Autodesk Inventor part; units mm, degrees
(part 3 of 3)
sketch "Sketch5" plane through (203.2, 0, 0) normal (0, 0, -1) x (-1, 0, 0)
  line L0 (0, 0) -> (203.2, 0) projected
  line L1 (0, 0) -> (0, -25.4) projected
  line L2 (203.2, -25.4) -> (0, -25.4) projected
  line L3 (203.2, 0) -> (203.2, -25.4) projected
  line L4 (18.6693, -4.254) -> (184.5307, -4.254) construction
  line L5 (184.5307, -4.254) -> (184.5307, -21.146) construction
  line L6 (184.5307, -21.146) -> (18.6693, -21.146) construction
  line L7 (18.6693, -21.146) -> (18.6693, -4.254) construction
  spline S0 degree 2 poles (29.2483, -14.4636) (29.2483, -15.1453) (28.7296, -16.1901) (28.2998, -16.531) knots 0 0 0 1 2 2 2
  spline S1 degree 2 poles (28.2998, -16.531) (27.7811, -16.9311) (26.6029, -17.272) (25.6692, -17.272) knots 0 0 0 1 2 2 2
  line L8 (25.6692, -17.272) -> (23.0461, -17.272)
  line L9 (23.0461, -17.272) -> (23.0461, -8.128)
  line L10 (23.0461, -8.128) -> (25.4692, -8.128)
  spline S2 degree 2 poles (25.4692, -8.128) (26.4473, -8.128) (27.4254, -8.254) (27.87, -8.4985) knots 0 0 0 1 2 2 2
  spline S3 degree 2 poles (27.87, -8.4985) (28.3665, -8.7579) (28.8185, -9.61) (28.8185, -10.188) knots 0 0 0 1 2 2 2
  spline S4 degree 2 poles (28.8185, -10.188) (28.8185, -10.8327) (28.1368, -11.8553) (27.5366, -12.1442) knots 0 0 0 1 2 2 2
  line L11 (27.5366, -12.1442) -> (27.5366, -12.1887)
  spline S5 degree 2 poles (27.5366, -12.1887) (28.3517, -12.411) (29.2483, -13.5892) (29.2483, -14.4636) knots 0 0 0 1 2 2 2
  spline S6 degree 2 poles (27.9812, -14.5155) (27.9812, -13.9968) (27.6848, -13.3299) (27.2402, -13.0927) knots 0 0 0 1 2 2 2
  spline S7 degree 2 poles (27.2402, -13.0927) (26.9512, -12.9445) (26.2694, -12.8556) (25.6396, -12.8556) knots 0 0 0 1 2 2 2
  line L12 (25.6396, -12.8556) -> (24.2613, -12.8556)
  line L13 (24.2613, -12.8556) -> (24.2613, -16.2346)
  line L14 (24.2613, -16.2346) -> (25.2469, -16.2346)
  spline S8 degree 2 poles (25.2469, -16.2346) (26.0471, -16.2346) (26.966, -16.0864) (27.3217, -15.8493) knots 0 0 0 1 2 2 2
  spline S9 degree 2 poles (27.3217, -15.8493) (27.6625, -15.6047) (27.9812, -14.9971) (27.9812, -14.5155) knots 0 0 0 1 2 2 2
  spline S10 degree 2 poles (27.5514, -10.3584) (27.5514, -10.0324) (27.3291, -9.5433) (27.0846, -9.4025) knots 0 0 0 1 2 2 2
  spline S11 degree 2 poles (27.0846, -9.4025) (26.7882, -9.2395) (26.0694, -9.1654) (25.4247, -9.1654) knots 0 0 0 1 2 2 2
  line L15 (25.4247, -9.1654) -> (24.2613, -9.1654)
  line L16 (24.2613, -9.1654) -> (24.2613, -11.8404)
  line L17 (24.2613, -11.8404) -> (25.6396, -11.8404)
  spline S12 degree 2 poles (25.6396, -11.8404) (26.2102, -11.8404) (26.7511, -11.7219) (27.0401, -11.5366) knots 0 0 0 1 2 2 2
  spline S13 degree 2 poles (27.0401, -11.5366) (27.3217, -11.3588) (27.5514, -10.7882) (27.5514, -10.3584) knots 0 0 0 1 2 2 2
  line L18 (29.4706, -17.272) -> (32.5532, -8.128)
  line L19 (32.5532, -8.128) -> (34.05, -8.128)
  line L20 (34.05, -8.128) -> (37.1326, -17.272)
  line L21 (37.1326, -17.272) -> (35.8506, -17.272)
  line L22 (35.8506, -17.272) -> (35.0207, -14.7155)
  line L23 (35.0207, -14.7155) -> (31.5306, -14.7155)
  line L24 (31.5306, -14.7155) -> (30.7007, -17.272)
  line L25 (30.7007, -17.272) -> (29.4706, -17.272)
  line L26 (34.6873, -13.6781) -> (33.2719, -9.3729)
  line L27 (33.2719, -9.3729) -> (31.864, -13.6781)
  line L28 (31.864, -13.6781) -> (34.6873, -13.6781)
  spline S14 degree 2 poles (40.5486, -17.435) (39.5557, -17.435) (38.1626, -17.0201) (37.5475, -16.7237) knots 0 0 0 1 2 2 2
  line L29 (37.5475, -16.7237) -> (37.5475, -15.1972)
  line L30 (37.5475, -15.1972) -> (37.6365, -15.1972)
  spline S15 degree 2 poles (37.6365, -15.1972) (38.2367, -15.7604) (39.7557, -16.3828) (40.4597, -16.3828) knots 0 0 0 1 2 2 2
  spline S16 degree 2 poles (40.4597, -16.3828) (41.4675, -16.3828) (42.4975, -15.5455) (42.4975, -14.8563) knots 0 0 0 1 2 2 2
  spline S17 degree 2 poles (42.4975, -14.8563) (42.4975, -14.308) (41.9565, -13.6263) (41.3711, -13.4558) knots 0 0 0 1 2 2 2
  spline S18 degree 2 poles (41.3711, -13.4558) (40.9488, -13.3373) (40.2448, -13.1742) (39.7187, -13.0409) knots 0 0 0 1 2 2 2
  spline S19 degree 2 poles (39.7187, -13.0409) (39.2444, -12.9149) (38.496, -12.537) (38.207, -12.2332) knots 0 0 0 1 2 2 2
  spline S20 degree 2 poles (38.207, -12.2332) (37.9255, -11.9294) (37.6142, -11.1142) (37.6142, -10.5807) knots 0 0 0 1 2 2 2
  spline S21 degree 2 poles (37.6142, -10.5807) (37.6142, -9.4692) (39.3482, -7.965) (40.6894, -7.965) knots 0 0 0 1 2 2 2
  spline S22 degree 2 poles (40.6894, -7.965) (41.46, -7.965) (42.8235, -8.2688) (43.4089, -8.5578) knots 0 0 0 1 2 2 2
  line L31 (43.4089, -8.5578) -> (43.4089, -10.0102)
  line L32 (43.4089, -10.0102) -> (43.32, -10.0102)
  spline S23 degree 2 poles (43.32, -10.0102) (42.8828, -9.61) (41.5193, -9.0172) (40.7709, -9.0172) knots 0 0 0 1 2 2 2
  spline S24 degree 2 poles (40.7709, -9.0172) (39.9262, -9.0172) (38.8814, -9.8101) (38.8814, -10.4548) knots 0 0 0 1 2 2 2
  spline S25 degree 2 poles (38.8814, -10.4548) (38.8814, -11.0327) (39.4964, -11.7219) (40.0744, -11.8775) knots 0 0 0 1 2 2 2
  spline S26 degree 2 poles (40.0744, -11.8775) (40.4597, -11.9812) (41.5786, -12.248) (41.9491, -12.3591) knots 0 0 0 1 2 2 2
  spline S27 degree 2 poles (41.9491, -12.3591) (42.8902, -12.6481) (43.7646, -13.8115) (43.7646, -14.6637) knots 0 0 0 1 2 2 2
  spline S28 degree 2 poles (43.7646, -14.6637) (43.7646, -15.2046) (43.3274, -16.242) (42.9346, -16.6051) knots 0 0 0 1 2 2 2
  spline S29 degree 2 poles (42.9346, -16.6051) (42.4975, -17.0052) (41.3859, -17.435) (40.5486, -17.435) knots 0 0 0 1 2 2 2
  line L33 (45.0021, -17.272) -> (45.0021, -8.128)
  line L34 (45.0021, -8.128) -> (50.7226, -8.128)
  line L35 (50.7226, -8.128) -> (50.7226, -9.2099)
  line L36 (50.7226, -9.2099) -> (46.2173, -9.2099)
  line L37 (46.2173, -9.2099) -> (46.2173, -11.7145)
  line L38 (46.2173, -11.7145) -> (50.4188, -11.7145)
  line L39 (50.4188, -11.7145) -> (50.4188, -12.7963)
  line L40 (50.4188, -12.7963) -> (46.2173, -12.7963)
  line L41 (46.2173, -12.7963) -> (46.2173, -16.1901)
  line L42 (46.2173, -16.1901) -> (50.7226, -16.1901)
  line L43 (50.7226, -16.1901) -> (50.7226, -17.272)
  line L44 (50.7226, -17.272) -> (45.0021, -17.272)
  line L45 (61.4524, -9.2099) -> (57.199, -9.2099)
  line L46 (57.199, -9.2099) -> (57.199, -11.7886)
  line L47 (57.199, -11.7886) -> (61.2745, -11.7886)
  line L48 (61.2745, -11.7886) -> (61.2745, -12.8704)
  line L49 (61.2745, -12.8704) -> (57.199, -12.8704)
  line L50 (57.199, -12.8704) -> (57.199, -17.272)
  line L51 (57.199, -17.272) -> (55.9837, -17.272)
  line L52 (55.9837, -17.272) -> (55.9837, -8.128)
  line L53 (55.9837, -8.128) -> (61.4524, -8.128)
  line L54 (61.4524, -8.128) -> (61.4524, -9.2099)
  spline S30 degree 2 poles (69.0106, -9.1728) (69.5293, -9.7804) (70.1073, -11.5589) (70.1073, -12.7) knots 0 0 0 1 2 2 2
  spline S31 degree 2 poles (70.1073, -12.7) (70.1073, -13.8115) (69.5441, -15.6121) (69.0106, -16.2198) knots 0 0 0 1 2 2 2
  spline S32 degree 2 poles (69.0106, -16.2198) (68.4474, -16.857) (66.958, -17.4647) (66.0614, -17.4647) knots 0 0 0 1 2 2 2
  spline S33 degree 2 poles (66.0614, -17.4647) (65.1352, -17.4647) (63.6531, -16.8348) (63.1122, -16.2198) knots 0 0 0 1 2 2 2
  spline S34 degree 2 poles (63.1122, -16.2198) (62.5861, -15.6121) (62.0229, -13.8263) (62.0229, -12.7) knots 0 0 0 1 2 2 2
  spline S35 degree 2 poles (62.0229, -12.7) (62.0229, -11.5514) (62.5935, -9.8027) (63.1196, -9.1728) knots 0 0 0 1 2 2 2
  spline S36 degree 2 poles (63.1196, -9.1728) (63.6531, -8.5652) (65.1426, -7.9353) (66.0614, -7.9353) knots 0 0 0 1 2 2 2
  spline S37 degree 2 poles (66.0614, -7.9353) (66.9951, -7.9353) (68.4919, -8.5874) (69.0106, -9.1728) knots 0 0 0 1 2 2 2
  spline S38 degree 2 poles (68.8402, -12.7) (68.8402, -11.796) (68.4474, -10.3955) (68.0918, -9.9361) knots 0 0 0 1 2 2 2
  spline S39 degree 2 poles (68.0918, -9.9361) (67.7287, -9.4618) (66.7061, -8.9876) (66.0688, -8.9876) knots 0 0 0 1 2 2 2
  spline S40 degree 2 poles (66.0688, -8.9876) (65.4093, -8.9876) (64.4164, -9.447) (64.0385, -9.9361) knots 0 0 0 1 2 2 2
  spline S41 degree 2 poles (64.0385, -9.9361) (63.6754, -10.4029) (63.2901, -11.8108) (63.2901, -12.7) knots 0 0 0 1 2 2 2
  spline S42 degree 2 poles (63.2901, -12.7) (63.2901, -14.5006) (64.8017, -16.4124) (66.0688, -16.4124) knots 0 0 0 1 2 2 2
  spline S43 degree 2 poles (66.0688, -16.4124) (67.3359, -16.4124) (68.8402, -14.5006) (68.8402, -12.7) knots 0 0 0 1 2 2 2
  spline S44 degree 2 poles (74.6348, -17.4647) (73.8271, -17.4647) (72.6267, -17.0423) (72.2043, -16.6199) knots 0 0 0 1 2 2 2
  spline S45 degree 2 poles (72.2043, -16.6199) (71.7227, -16.1457) (71.33, -14.8119) (71.33, -13.8337) knots 0 0 0 1 2 2 2
  line L55 (71.33, -13.8337) -> (71.33, -8.128)
  line L56 (71.33, -8.128) -> (72.5452, -8.128)
  line L57 (72.5452, -8.128) -> (72.5452, -13.8337)
  spline S46 degree 2 poles (72.5452, -13.8337) (72.5452, -14.471) (72.7082, -15.3306) (72.9379, -15.6788) knots 0 0 0 1 2 2 2
  spline S47 degree 2 poles (72.9379, -15.6788) (73.1825, -16.0493) (74.0272, -16.4273) (74.6348, -16.4273) knots 0 0 0 1 2 2 2
  spline S48 degree 2 poles (74.6348, -16.4273) (75.2054, -16.4273) (76.0946, -16.0493) (76.3391, -15.6788) knots 0 0 0 1 2 2 2
  spline S49 degree 2 poles (76.3391, -15.6788) (76.5689, -15.3306) (76.7319, -14.4784) (76.7319, -13.8634) knots 0 0 0 1 2 2 2
  line L58 (76.7319, -13.8634) -> (76.7319, -8.128)
  line L59 (76.7319, -8.128) -> (77.9471, -8.128)
  line L60 (77.9471, -8.128) -> (77.9471, -13.8337)
  spline S50 degree 2 poles (77.9471, -13.8337) (77.9471, -14.7896) (77.5618, -16.1531) (77.0727, -16.6199) knots 0 0 0 1 2 2 2
  spline S51 degree 2 poles (77.0727, -16.6199) (76.6355, -17.0497) (75.4796, -17.4647) (74.6348, -17.4647) knots 0 0 0 1 2 2 2
  line L61 (86.7651, -17.272) -> (85.1867, -17.272)
  line L62 (85.1867, -17.272) -> (82.2968, -13.6337)
  line L63 (82.2968, -13.6337) -> (80.9037, -13.6337)
  line L64 (80.9037, -13.6337) -> (80.9037, -17.272)
  line L65 (80.9037, -17.272) -> (79.6885, -17.272)
  line L66 (79.6885, -17.272) -> (79.6885, -8.128)
  line L67 (79.6885, -8.128) -> (82.0449, -8.128)
  spline S52 degree 2 poles (82.0449, -8.128) (82.8303, -8.128) (83.89, -8.2984) (84.3716, -8.6097) knots 0 0 0 1 2 2 2
  spline S53 degree 2 poles (84.3716, -8.6097) (84.8533, -8.9209) (85.409, -9.8916) (85.409, -10.6104) knots 0 0 0 1 2 2 2
  spline S54 degree 2 poles (85.409, -10.6104) (85.409, -11.6107) (84.3865, -12.9668) (83.5121, -13.2928) knots 0 0 0 1 2 2 2
  line L68 (83.5121, -13.2928) -> (86.7651, -17.272)
  spline S55 degree 2 poles (84.1419, -10.7067) (84.1419, -10.3066) (83.8603, -9.6915) (83.5639, -9.4914) knots 0 0 0 1 2 2 2
  spline S56 degree 2 poles (83.5639, -9.4914) (83.3046, -9.321) (82.6155, -9.1802) (82.1116, -9.1802) knots 0 0 0 1 2 2 2
  line L69 (82.1116, -9.1802) -> (80.9037, -9.1802)
  line L70 (80.9037, -9.1802) -> (80.9037, -12.6185)
  line L71 (80.9037, -12.6185) -> (81.9708, -12.6185)
  spline S57 degree 2 poles (81.9708, -12.6185) (82.4969, -12.6185) (83.3342, -12.4332) (83.6232, -12.1442) knots 0 0 0 1 2 2 2
  spline S58 degree 2 poles (83.6232, -12.1442) (83.89, -11.8923) (84.1419, -11.1809) (84.1419, -10.7067) knots 0 0 0 1 2 2 2
  line L72 (90.6776, -17.272) -> (87.1356, -17.272)
  line L73 (87.1356, -17.272) -> (87.1356, -16.3383)
  line L74 (87.1356, -16.3383) -> (88.299, -16.3383)
  line L75 (88.299, -16.3383) -> (88.299, -9.0617)
  line L76 (88.299, -9.0617) -> (87.1356, -9.0617)
  line L77 (87.1356, -9.0617) -> (87.1356, -8.128)
  line L78 (87.1356, -8.128) -> (90.6776, -8.128)
  line L79 (90.6776, -8.128) -> (90.6776, -9.0617)
  line L80 (90.6776, -9.0617) -> (89.5142, -9.0617)
  line L81 (89.5142, -9.0617) -> (89.5142, -16.3383)
  line L82 (89.5142, -16.3383) -> (90.6776, -16.3383)
  line L83 (90.6776, -16.3383) -> (90.6776, -17.272)
  line L84 (92.1818, -17.272) -> (92.1818, -8.128)
  line L85 (92.1818, -8.128) -> (97.9024, -8.128)
  line L86 (97.9024, -8.128) -> (97.9024, -9.2099)
  line L87 (97.9024, -9.2099) -> (93.3971, -9.2099)
  line L88 (93.3971, -9.2099) -> (93.3971, -11.7145)
  line L89 (93.3971, -11.7145) -> (97.5986, -11.7145)
  line L90 (97.5986, -11.7145) -> (97.5986, -12.7963)
  line L91 (97.5986, -12.7963) -> (93.3971, -12.7963)
  line L92 (93.3971, -12.7963) -> (93.3971, -16.1901)
  line L93 (93.3971, -16.1901) -> (97.9024, -16.1901)
  line L94 (97.9024, -16.1901) -> (97.9024, -17.272)
  line L95 (97.9024, -17.272) -> (92.1818, -17.272)
  line L96 (106.3128, -17.272) -> (104.7345, -17.272)
  line L97 (104.7345, -17.272) -> (101.8445, -13.6337)
  line L98 (101.8445, -13.6337) -> (100.4514, -13.6337)
  line L99 (100.4514, -13.6337) -> (100.4514, -17.272)
  line L100 (100.4514, -17.272) -> (99.2362, -17.272)
  line L101 (99.2362, -17.272) -> (99.2362, -8.128)
  line L102 (99.2362, -8.128) -> (101.5926, -8.128)
  spline S59 degree 2 poles (101.5926, -8.128) (102.3781, -8.128) (103.4377, -8.2984) (103.9193, -8.6097) knots 0 0 0 1 2 2 2
  spline S60 degree 2 poles (103.9193, -8.6097) (104.401, -8.9209) (104.9568, -9.8916) (104.9568, -10.6104) knots 0 0 0 1 2 2 2
  spline S61 degree 2 poles (104.9568, -10.6104) (104.9568, -11.6107) (103.9342, -12.9668) (103.0598, -13.2928) knots 0 0 0 1 2 2 2
  line L103 (103.0598, -13.2928) -> (106.3128, -17.272)
  spline S62 degree 2 poles (103.6896, -10.7067) (103.6896, -10.3066) (103.4081, -9.6915) (103.1117, -9.4914) knots 0 0 0 1 2 2 2
  spline S63 degree 2 poles (103.1117, -9.4914) (102.8523, -9.321) (102.1632, -9.1802) (101.6593, -9.1802) knots 0 0 0 1 2 2 2
  line L104 (101.6593, -9.1802) -> (100.4514, -9.1802)
  line L105 (100.4514, -9.1802) -> (100.4514, -12.6185)
  line L106 (100.4514, -12.6185) -> (101.5185, -12.6185)
  spline S64 degree 2 poles (101.5185, -12.6185) (102.0446, -12.6185) (102.8819, -12.4332) (103.1709, -12.1442) knots 0 0 0 1 2 2 2
  spline S65 degree 2 poles (103.1709, -12.1442) (103.4377, -11.8923) (103.6896, -11.1809) (103.6896, -10.7067) knots 0 0 0 1 2 2 2
  line L107 (113.1004, -17.272) -> (113.1004, -9.2099)
  line L108 (113.1004, -9.2099) -> (110.0326, -9.2099)
  line L109 (110.0326, -9.2099) -> (110.0326, -8.128)
  line L110 (110.0326, -8.128) -> (117.3834, -8.128)
  line L111 (117.3834, -8.128) -> (117.3834, -9.2099)
  line L112 (117.3834, -9.2099) -> (114.3156, -9.2099)
  line L113 (114.3156, -9.2099) -> (114.3156, -17.272)
  line L114 (114.3156, -17.272) -> (113.1004, -17.272)
  line L115 (125.3863, -17.272) -> (123.8079, -17.272)
  line L116 (123.8079, -17.272) -> (120.918, -13.6337)
  line L117 (120.918, -13.6337) -> (119.5249, -13.6337)
  line L118 (119.5249, -13.6337) -> (119.5249, -17.272)
  line L119 (119.5249, -17.272) -> (118.3097, -17.272)
  line L120 (118.3097, -17.272) -> (118.3097, -8.128)
  line L121 (118.3097, -8.128) -> (120.6661, -8.128)
  spline S66 degree 2 poles (120.6661, -8.128) (121.4515, -8.128) (122.5112, -8.2984) (122.9928, -8.6097) knots 0 0 0 1 2 2 2
  spline S67 degree 2 poles (122.9928, -8.6097) (123.4745, -8.9209) (124.0302, -9.8916) (124.0302, -10.6104) knots 0 0 0 1 2 2 2
  spline S68 degree 2 poles (124.0302, -10.6104) (124.0302, -11.6107) (123.0076, -12.9668) (122.1332, -13.2928) knots 0 0 0 1 2 2 2
  line L122 (122.1332, -13.2928) -> (125.3863, -17.272)
  spline S69 degree 2 poles (122.7631, -10.7067) (122.7631, -10.3066) (122.4815, -9.6915) (122.1851, -9.4914) knots 0 0 0 1 2 2 2
  spline S70 degree 2 poles (122.1851, -9.4914) (121.9258, -9.321) (121.2366, -9.1802) (120.7327, -9.1802) knots 0 0 0 1 2 2 2
  line L123 (120.7327, -9.1802) -> (119.5249, -9.1802)
  line L124 (119.5249, -9.1802) -> (119.5249, -12.6185)
  line L125 (119.5249, -12.6185) -> (120.592, -12.6185)
  spline S71 degree 2 poles (120.592, -12.6185) (121.1181, -12.6185) (121.9554, -12.4332) (122.2444, -12.1442) knots 0 0 0 1 2 2 2
  spline S72 degree 2 poles (122.2444, -12.1442) (122.5112, -11.8923) (122.7631, -11.1809) (122.7631, -10.7067) knots 0 0 0 1 2 2 2
  line L126 (125.1269, -17.272) -> (128.2095, -8.128)
  line L127 (128.2095, -8.128) -> (129.7063, -8.128)
  line L128 (129.7063, -8.128) -> (132.7889, -17.272)
  line L129 (132.7889, -17.272) -> (131.507, -17.272)
  line L130 (131.507, -17.272) -> (130.677, -14.7155)
  line L131 (130.677, -14.7155) -> (127.1869, -14.7155)
  line L132 (127.1869, -14.7155) -> (126.357, -17.272)
  line L133 (126.357, -17.272) -> (125.1269, -17.272)
  line L134 (130.3436, -13.6781) -> (128.9283, -9.3729)
  line L135 (128.9283, -9.3729) -> (127.5204, -13.6781)
  line L136 (127.5204, -13.6781) -> (130.3436, -13.6781)
  line L137 (140.1989, -17.272) -> (138.8355, -17.272)
  line L138 (138.8355, -17.272) -> (134.7896, -9.3877)
  line L139 (134.7896, -9.3877) -> (134.7896, -17.272)
  line L140 (134.7896, -17.272) -> (133.6559, -17.272)
  line L141 (133.6559, -17.272) -> (133.6559, -8.128)
  line L142 (133.6559, -8.128) -> (135.3824, -8.128)
  line L143 (135.3824, -8.128) -> (139.0652, -15.3676)
  line L144 (139.0652, -15.3676) -> (139.0652, -8.128)
  line L145 (139.0652, -8.128) -> (140.1989, -8.128)
  line L146 (140.1989, -8.128) -> (140.1989, -17.272)
  spline S73 degree 2 poles (144.6005, -17.435) (143.6076, -17.435) (142.2145, -17.0201) (141.5994, -16.7237) knots 0 0 0 1 2 2 2
  line L147 (141.5994, -16.7237) -> (141.5994, -15.1972)
  line L148 (141.5994, -15.1972) -> (141.6884, -15.1972)
  spline S74 degree 2 poles (141.6884, -15.1972) (142.2886, -15.7604) (143.8076, -16.3828) (144.5116, -16.3828) knots 0 0 0 1 2 2 2
  spline S75 degree 2 poles (144.5116, -16.3828) (145.5194, -16.3828) (146.5494, -15.5455) (146.5494, -14.8563) knots 0 0 0 1 2 2 2
  spline S76 degree 2 poles (146.5494, -14.8563) (146.5494, -14.308) (146.0084, -13.6263) (145.423, -13.4558) knots 0 0 0 1 2 2 2
  spline S77 degree 2 poles (145.423, -13.4558) (145.0007, -13.3373) (144.2967, -13.1742) (143.7706, -13.0409) knots 0 0 0 1 2 2 2
  spline S78 degree 2 poles (143.7706, -13.0409) (143.2963, -12.9149) (142.5479, -12.537) (142.2589, -12.2332) knots 0 0 0 1 2 2 2
  spline S79 degree 2 poles (142.2589, -12.2332) (141.9774, -11.9294) (141.6661, -11.1142) (141.6661, -10.5807) knots 0 0 0 1 2 2 2
  spline S80 degree 2 poles (141.6661, -10.5807) (141.6661, -9.4692) (143.4001, -7.965) (144.7413, -7.965) knots 0 0 0 1 2 2 2
  spline S81 degree 2 poles (144.7413, -7.965) (145.5119, -7.965) (146.8754, -8.2688) (147.4608, -8.5578) knots 0 0 0 1 2 2 2
  line L149 (147.4608, -8.5578) -> (147.4608, -10.0102)
  line L150 (147.4608, -10.0102) -> (147.3719, -10.0102)
  spline S82 degree 2 poles (147.3719, -10.0102) (146.9347, -9.61) (145.5712, -9.0172) (144.8228, -9.0172) knots 0 0 0 1 2 2 2
  spline S83 degree 2 poles (144.8228, -9.0172) (143.9781, -9.0172) (142.9333, -9.8101) (142.9333, -10.4548) knots 0 0 0 1 2 2 2
  spline S84 degree 2 poles (142.9333, -10.4548) (142.9333, -11.0327) (143.5483, -11.7219) (144.1263, -11.8775) knots 0 0 0 1 2 2 2
  spline S85 degree 2 poles (144.1263, -11.8775) (144.5116, -11.9812) (145.6305, -12.248) (146.001, -12.3591) knots 0 0 0 1 2 2 2
  spline S86 degree 2 poles (146.001, -12.3591) (146.9421, -12.6481) (147.8165, -13.8115) (147.8165, -14.6637) knots 0 0 0 1 2 2 2
  spline S87 degree 2 poles (147.8165, -14.6637) (147.8165, -15.2046) (147.3793, -16.242) (146.9865, -16.6051) knots 0 0 0 1 2 2 2
  spline S88 degree 2 poles (146.9865, -16.6051) (146.5494, -17.0052) (145.4378, -17.435) (144.6005, -17.435) knots 0 0 0 1 2 2 2
  line L151 (154.5226, -9.2099) -> (150.2692, -9.2099)
  line L152 (150.2692, -9.2099) -> (150.2692, -11.7886)
  line L153 (150.2692, -11.7886) -> (154.3447, -11.7886)
  line L154 (154.3447, -11.7886) -> (154.3447, -12.8704)
  line L155 (154.3447, -12.8704) -> (150.2692, -12.8704)
  line L156 (150.2692, -12.8704) -> (150.2692, -17.272)
  line L157 (150.2692, -17.272) -> (149.054, -17.272)
  line L158 (149.054, -17.272) -> (149.054, -8.128)
  line L159 (149.054, -8.128) -> (154.5226, -8.128)
  line L160 (154.5226, -8.128) -> (154.5226, -9.2099)
  spline S89 degree 2 poles (162.0808, -9.1728) (162.5995, -9.7804) (163.1775, -11.5589) (163.1775, -12.7) knots 0 0 0 1 2 2 2
  spline S90 degree 2 poles (163.1775, -12.7) (163.1775, -13.8115) (162.6143, -15.6121) (162.0808, -16.2198) knots 0 0 0 1 2 2 2
  spline S91 degree 2 poles (162.0808, -16.2198) (161.5177, -16.857) (160.0282, -17.4647) (159.1316, -17.4647) knots 0 0 0 1 2 2 2
  spline S92 degree 2 poles (159.1316, -17.4647) (158.2054, -17.4647) (156.7234, -16.8348) (156.1824, -16.2198) knots 0 0 0 1 2 2 2
  spline S93 degree 2 poles (156.1824, -16.2198) (155.6563, -15.6121) (155.0931, -13.8263) (155.0931, -12.7) knots 0 0 0 1 2 2 2
  spline S94 degree 2 poles (155.0931, -12.7) (155.0931, -11.5514) (155.6637, -9.8027) (156.1898, -9.1728) knots 0 0 0 1 2 2 2
  spline S95 degree 2 poles (156.1898, -9.1728) (156.7234, -8.5652) (158.2128, -7.9353) (159.1316, -7.9353) knots 0 0 0 1 2 2 2
  spline S96 degree 2 poles (159.1316, -7.9353) (160.0653, -7.9353) (161.5621, -8.5874) (162.0808, -9.1728) knots 0 0 0 1 2 2 2
  spline S97 degree 2 poles (161.9104, -12.7) (161.9104, -11.796) (161.5177, -10.3955) (161.162, -9.9361) knots 0 0 0 1 2 2 2
  spline S98 degree 2 poles (161.162, -9.9361) (160.7989, -9.4618) (159.7763, -8.9876) (159.139, -8.9876) knots 0 0 0 1 2 2 2
  spline S99 degree 2 poles (159.139, -8.9876) (158.4795, -8.9876) (157.4866, -9.447) (157.1087, -9.9361) knots 0 0 0 1 2 2 2
  spline S100 degree 2 poles (157.1087, -9.9361) (156.7456, -10.4029) (156.3603, -11.8108) (156.3603, -12.7) knots 0 0 0 1 2 2 2
  spline S101 degree 2 poles (156.3603, -12.7) (156.3603, -14.5006) (157.8719, -16.4124) (159.139, -16.4124) knots 0 0 0 1 2 2 2
  spline S102 degree 2 poles (159.139, -16.4124) (160.4061, -16.4124) (161.9104, -14.5006) (161.9104, -12.7) knots 0 0 0 1 2 2 2
  line L161 (171.5879, -17.272) -> (170.0096, -17.272)
  line L162 (170.0096, -17.272) -> (167.1197, -13.6337)
  line L163 (167.1197, -13.6337) -> (165.7266, -13.6337)
  line L164 (165.7266, -13.6337) -> (165.7266, -17.272)
  line L165 (165.7266, -17.272) -> (164.5113, -17.272)
  line L166 (164.5113, -17.272) -> (164.5113, -8.128)
  line L167 (164.5113, -8.128) -> (166.8677, -8.128)
  spline S103 degree 2 poles (166.8677, -8.128) (167.6532, -8.128) (168.7128, -8.2984) (169.1945, -8.6097) knots 0 0 0 1 2 2 2
  spline S104 degree 2 poles (169.1945, -8.6097) (169.6761, -8.9209) (170.2319, -9.8916) (170.2319, -10.6104) knots 0 0 0 1 2 2 2
  spline S105 degree 2 poles (170.2319, -10.6104) (170.2319, -11.6107) (169.2093, -12.9668) (168.3349, -13.2928) knots 0 0 0 1 2 2 2
  line L168 (168.3349, -13.2928) -> (171.5879, -17.272)
  spline S106 degree 2 poles (168.9648, -10.7067) (168.9648, -10.3066) (168.6832, -9.6915) (168.3868, -9.4914) knots 0 0 0 1 2 2 2
  spline S107 degree 2 poles (168.3868, -9.4914) (168.1274, -9.321) (167.4383, -9.1802) (166.9344, -9.1802) knots 0 0 0 1 2 2 2
  line L169 (166.9344, -9.1802) -> (165.7266, -9.1802)
  line L170 (165.7266, -9.1802) -> (165.7266, -12.6185)
  line L171 (165.7266, -12.6185) -> (166.7936, -12.6185)
  spline S108 degree 2 poles (166.7936, -12.6185) (167.3197, -12.6185) (168.1571, -12.4332) (168.446, -12.1442) knots 0 0 0 1 2 2 2
  spline S109 degree 2 poles (168.446, -12.1442) (168.7128, -11.8923) (168.9648, -11.1809) (168.9648, -10.7067) knots 0 0 0 1 2 2 2
  line L172 (180.1539, -17.272) -> (178.9387, -17.272)
  line L173 (178.9387, -17.272) -> (178.9387, -9.3951)
  line L174 (178.9387, -9.3951) -> (176.5526, -14.7526)
  line L175 (176.5526, -14.7526) -> (175.8116, -14.7526)
  line L176 (175.8116, -14.7526) -> (173.4478, -9.3951)
  line L177 (173.4478, -9.3951) -> (173.4478, -17.272)
  line L178 (173.4478, -17.272) -> (172.3141, -17.272)
  line L179 (172.3141, -17.272) -> (172.3141, -8.128)
  line L180 (172.3141, -8.128) -> (173.9739, -8.128)
  line L181 (173.9739, -8.128) -> (176.2562, -13.2187)
  line L182 (176.2562, -13.2187) -> (178.4644, -8.128)
  line L183 (178.4644, -8.128) -> (180.1539, -8.128)
  line L184 (180.1539, -8.128) -> (180.1539, -17.272)
  dimension "d30" = 203.2
  dimension "d31" = 25.4
  dimension "d32" = 165.8615
  dimension "d33" = 16.892
  dimension "d34" = 18.6693
  dimension "d35" = 4.254
  constraints: 2 other
  measures "d30" distance of L0.start L0.end
  measures "d31" distance of L0.start L1.end
  measures "d32" distance of L4.start L4.end
  measures "d33" distance of L6.end L4.start
  measures "d34" distance between parallel lines of L1 L7
  measures "d35" distance between parallel lines of L0 L4
extrude "Extrusion5" cut sketch "Sketch5" against normal blind 5.08 contours S0 S1 L8 L9 L10 S2 S3 S4 L11 S5 | L18 L19 L20 L21 L22 L23 L24 L25 | S14 L29 L30 S15 S16 S17 S18 S19 S20 S21 S22 L31 L32 S23 S24 S25 S26 S27 S28 S29 | L33 L34 L35 L36 L37 L38 L39 L40 L41 L42 L43 L44 | L45 L46 L47 L48 L49 L50 L51 L52 L53 L54 | S30 S31 S32 S33 S34 S35 S36 S37 | S44 S45 L55 L56 L57 S46 S47 S48 S49 L58 L59 L60 S50 S51 | L61 L62 L63 L64 L65 L66 L67 S52 S53 S54 L68 | L72 L73 L74 L75 L76 L77 L78 L79 L80 L81 L82 L83 | L84 L85 L86 L87 L88 L89 L90 L91 L92 L93 L94 L95 | L96 L97 L98 L99 L100 L101 L102 S59 S60 S61 L103 | L107 L108 L109 L110 L111 L112 L113 L114 | L115 L126 L122 | L122 L126 L127 L128 L129 L130 L131 L132 L133 | L115 L116 L117 L118 L119 L120 L121 S66 S67 S68 L122 L126 | L137 L138 L139 L140 L141 L142 L143 L144 L145 L146 | S73 L147 L148 S74 S75 S76 S77 S78 S79 S80 S81 L149 L150 S82 S83 S84 S85 S86 S87 S88 | L151 L152 L153 L154 L155 L156 L157 L158 L159 L160 | S89 S90 S91 S92 S93 S94 S95 S96 | L161 L162 L163 L164 L165 L166 L167 S103 S104 S105 L168 | L172 L173 L174 L175 L176 L177 L178 L179 L180 L181 L182 L183 L184
equation "\"d6\" = 0.5 * d3 - 0.5 * d5"
equation "\"d7\" = 0.5 * d2 - 0.5 * d4"
equation "\"d16\" = 0.5 * d11 - 0.5 * d15"
equation "\"d17\" = 0.5 * d11 - 0.5 * d13"
equation "\"d18\" = -0.333333 * d12 + 0.333333 * d10 - 0.333333 * d14"
equation "\"d19\" = d18"
equation "\"d26\" = 0.5 * d22 - 0.5 * d24"
equation "\"d27\" = 0.5 * d23 - 0.5 * d25"
equation "\"d34\" = 0.5 * d30 - 0.5 * d32"
equation "\"d35\" = 0.5 * d31 - 0.5 * d33"
body "Solid1"
